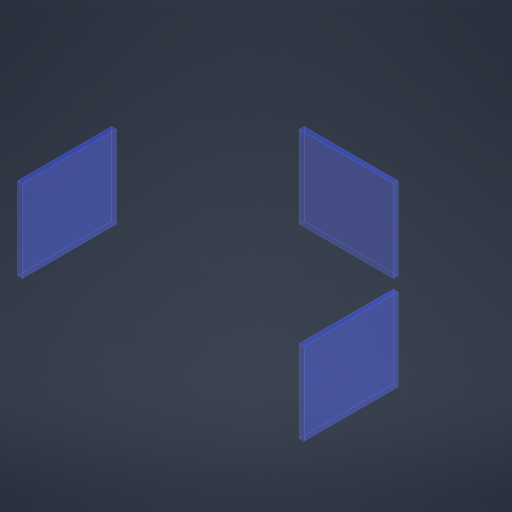
# Autodesk Inventor part: sklo
Saved by Autodesk Inventor 2023 (Build 270158000, 158)
## iProperties
Created: 2022-10-19
Part Number: sklo
Material: Sklo
Document SubType Name: Modeling
Designer: matej
Mass: 18.312 g
Surface Area: 93 cm^2
Volume: 8.4 cm^3
Density: 2.18 g/cm^3
Appearance: Čirá – modrá
Author: matej
Autodesk Inventor part; units mm, degrees
ref_plane "YZ Plane" through (0, 0, 0) normal (1, 0, 0) x (0, 1, 0)
ref_plane "XZ Plane" through (0, 0, 0) normal (0, 1, 0) x (-1, 0, 0)
ref_plane "XY Plane" through (0, 0, 0) normal (0, 0, 1) x (1, 0, 0)
sketch "Náčrt2" plane through (0, 0, 0) normal (0, 1, 0) x (-1, 0, 0)
  line L0 (61, -20) -> (59, -20)
  line L1 (59, -20) -> (59, 20)
  line L2 (59, 20) -> (61, 20)
  line L3 (61, 20) -> (61, -20)
  line L4 (75, -75) -> (75, 75)
  line L5 (45, 45) -> (45, -45)
  line L6 (75, 15) -> (45, 15)
  line L7 (75, -15) -> (45, -15)
  line L8 (0, 17.5556) -> (0, -18.0256) construction
  line L9 (-61, -20) -> (-59, -20)
  line L10 (-59, -20) -> (-59, 20)
  line L11 (-59, 20) -> (-61, 20)
  line L12 (-61, 20) -> (-61, -20)
  line L13 (-75, 15) -> (-45, 15)
  line L14 (-75, -15) -> (-45, -15)
  line L15 (75, 75) -> (-75, 75) construction
  line L16 (0, 0) -> (-75, 75) construction
  line L17 (-20, 59) -> (-20, 61)
  line L18 (-15, 75) -> (-15, 45)
  line L19 (20, 59) -> (-20, 59)
  line L20 (20, 61) -> (20, 59)
  line L21 (-20, 61) -> (20, 61)
  line L22 (15, 75) -> (15, 45)
  line L23 (20, 0) -> (-37.5, 0) construction
  line L24 (-20, -59) -> (-20, -61)
  line L25 (-15, -75) -> (-15, -45)
  line L26 (20, -59) -> (-20, -59)
  line L27 (20, -61) -> (20, -59)
  line L28 (-20, -61) -> (20, -61)
  line L29 (15, -75) -> (15, -45)
  point P0 (59, 0)
  point P1 (60, 20)
  point P2 (60, -20)
  point P3 (-59, 0)
  point P4 (-60, 20)
  point P5 (-60, -20)
  point P6 (0, 59)
  point P7 (20, 60)
  point P8 (-20, 60)
  point P9 (0, -59)
  point P10 (-20, -60)
  point P11 (20, -60)
  dimension "d0" = 2
  dimension "d1" = 14
  dimension "d2" = 14
  dimension "d3" = 5
  dimension "d4" = 5
  constraints: 60 end point, 33 symmetric about line, 3 midpoint, 2 horizontal, 2 parallel, 1 perpendicular, 1 vertical
  measures "d0" distance from line of L3 point (59, 0)
  measures "d1" distance between parallel lines of L4 L3
  measures "d2" distance between parallel lines of L5 L1
  measures "d3" distance from line of L6 point (60, 20)
  measures "d4" distance from line of L7 point (60, -20)
extrude "Vysunutí1" add sketch "Náčrt2" along normal blind 35 contours L0 L1 L7 L3 | L7 L1 L6 L3 | L6 L1 L2 L3 | L12 L14 L10 L9 | L12 L13 L10 L14 | L12 L11 L10 L13 | L26 L25 L28 L24 | L26 L29 L28 L25 | L26 L27 L28 L29
